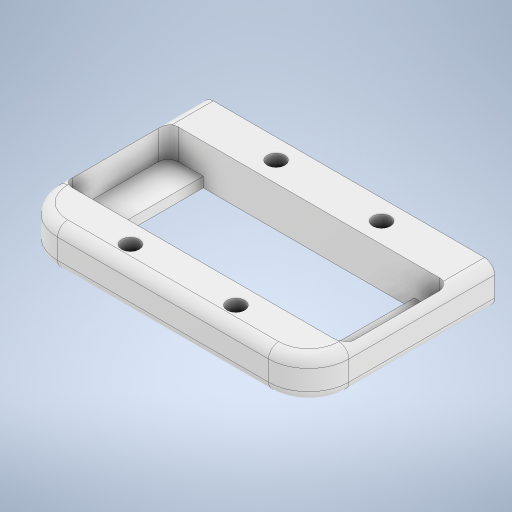
# Autodesk Inventor part: CoxaServoCutout
Saved by Autodesk Inventor 2024 (Build 280153000, 153)
## iProperties
Created: 2026-02-24
Part Number: CoxaServoCutout
Material: Generic
Document SubType Name: Modeling
Designer: Liam
Density: 1 g/cm^3
Appearance: Default
Author: Liam
Autodesk Inventor part; units mm, degrees
ref_plane "YZ Plane" through (0, 0, 0) normal (1, 0, 0) x (0, 1, 0)
ref_plane "XZ Plane" through (0, 0, 0) normal (0, 1, 0) x (-1, 0, 0)
ref_plane "XY Plane" through (0, 0, 0) normal (0, 0, 1) x (1, 0, 0)
sketch "Sketch1" plane through (0, 0, 0) normal (0, 1, 0) x (-1, 0, 0)
  line L0 (21, 10.5) -> (-21, 10.5)
  line L1 (-21, 10.5) -> (-21, -10.5)
  line L2 (-21, -10.5) -> (21, -10.5)
  line L3 (21, -10.5) -> (21, 10.5)
  line L4 (21, 10.5) -> (-21, -10.5) construction
  line L5 (-21, 10.5) -> (21, -10.5) construction
  line L6 (-29, 18.5) -> (29, 18.5)
  line L7 (29, 18.5) -> (29, -18.5)
  line L8 (29, -18.5) -> (-29, -18.5)
  line L9 (-29, -18.5) -> (-29, 18.5)
  circle A0 centre (10.5, 14.5) radius 1.75
  line L10 (0, 10.5) -> (0, -10.5) construction
  line L11 (-21, 0) -> (21, 0) construction
  circle A1 centre (10.5, -14.5) radius 1.75
  circle A2 centre (-10.5, 14.5) radius 1.75
  circle A3 centre (-10.5, -14.5) radius 1.75
  line L12 (-21, 10.5) -> (-28, 10.5)
  line L13 (-28, 10.5) -> (-28, -10.5)
  line L14 (-28, -10.5) -> (-21, -10.5)
  line L15 (-21, -10.5) -> (-21, 10.5)
  line L16 (21, 10.5) -> (28, 10.5)
  line L17 (28, 10.5) -> (28, -10.5)
  line L18 (28, -10.5) -> (21, -10.5)
  point P0 (0, 0)
  dimension "d0" = 21
  dimension "d1" = 42
  dimension "d2" = 8
  dimension "d3" = 3.5
  dimension "d4" = 10.5
  dimension "d5" = 4
  dimension "d6" = 7
  dimension "d7" = 21
  constraints: 38 end point, 6 midpoint, 6 parallel, 6 symmetric about line, 4 centre point, 3 perpendicular, 2 horizontal, 6 other
  measures "d0" distance of L2.end L0.start
  measures "d1" distance of L0.start L0.end
  measures "d2" distance between parallel lines of L0 L6
  measures "d3" diameter of A0
  measures "d4" distance from line of L10 A0.centre
  measures "d5" distance from line of L0 A0.centre
  measures "d6" distance of L13.end L14.end
  measures "d7" distance of L12.end L13.end
extrude "Extrusion1" add sketch "Sketch1" along normal blind 8
extrude "Extrusion2" add sketch "Sketch1" along normal blind 2 contours L16 L17 L18 L3 | L1 L14 L13 L12
fillet "Fillet1" radius 8 2 edges at (-29, 4, 18.5) (29, 4, 18.5)
fillet "Fillet2" radius 2 4 edges at (-28, 5, 10.5) (-28, 5, -10.5) (28, 5, 10.5) (28, 5, -10.5)
fillet "Fillet3" radius 2 10 edges at (-26.6569, 0, 16.1569) (0, 0, 18.5) (26.6569, 0, 16.1569) (29, 0, -4) (-29, 0, -4) (-26.6569, 8, 16.1569) (0, 8, 18.5) (26.6569, 8, 16.1569) (29, 8, -4) (-29, 8, -4)
equation "\"d0\" = MountWidth"
equation "\"d1\" = MountLength"
equation "\"d2\" = MountThickness"
equation "\"d3\" = THROUGH_DIAMETER"
equation "\"d4\" = 0.25 * MountLength"
equation "\"d5\" = 0.5 * MountThickness"
equation "\"d7\" = MountWidth"
equation "\"d8\" = OUTER_HEIGHT"
equation "\"d12\" = OUTER_FILLET"
equation "\"d13\" = INNER_FILLET"
equation "\"d14\" = PART_FILLET"
equation "\"MountWidth\" = 21"
equation "\"MountLength\" = 42"
equation "\"MountThickness\" = 8"
equation "\"THROUGH_DIAMETER\" = 3.5"
equation "\"OUTER_HEIGHT\" = 8"
equation "\"OUTER_FILLET\" = 8"
equation "\"INNER_FILLET\" = 2"
equation "\"PART_FILLET\" = 2"
body "Solid1"
